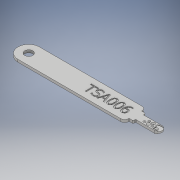
# Autodesk Inventor part: TSA006
Saved by Autodesk Inventor 2018 (Build 220112000, 112)
## iProperties
Created: 2018-08-22
Part Number: TSA006
Material: Generic
Document SubType Name: Modeling
Designer: Fatts
Density: 1 g/cm^3
Appearance: Default
Author: Fatts
Autodesk Inventor part; units mm, degrees
ref_plane "YZ Plane" through (0, 0, 0) normal (1, 0, 0) x (0, 1, 0)
ref_plane "XZ Plane" through (0, 0, 0) normal (0, 1, 0) x (-1, 0, 0)
ref_plane "XY Plane" through (0, 0, 0) normal (0, 0, 1) x (1, 0, 0)
sketch "Sketch1" plane through (0, 0, 0) normal (0, 1, 0) x (-1, 0, 0)
  line L0 (3.048, 7.366) -> (3.048, -7.366)
  line L1 (-3.048, 7.366) -> (-3.048, -7.366)
  line L2 (3.048, 0) -> (-3.048, 0) construction
  line L3 (3.048, -7.366) -> (-3.048, -7.366) construction
  arc A0 (-3.048, -7.366) -> (3.048, -7.366) centre (0, -6.7917) ccw
  line L4 (4.9022, 8.636) -> (4.9022, 10.6426)
  line L5 (-4.9022, 10.6426) -> (-4.9022, 8.636)
  line L6 (4.9022, 9.6393) -> (-4.9022, 9.6393) construction
  line L7 (0, 0) -> (0, 9.6393) construction
  line L8 (-4.0132, 7.747) -> (-3.429, 7.747)
  line L9 (3.429, 7.747) -> (4.0132, 7.747)
  arc A1 (4.0132, 7.747) -> (4.9022, 8.636) centre (4.0132, 8.636) ccw
  arc A2 (-4.9022, 8.636) -> (-4.0132, 7.747) centre (-4.0132, 8.636) ccw
  arc A3 (3.429, 7.747) -> (3.048, 7.366) centre (3.429, 7.366) ccw
  arc A4 (-3.048, 7.366) -> (-3.429, 7.747) centre (-3.429, 7.366) ccw
  line L10 (8.3947, 102.9462) -> (8.3947, 11.0236)
  line L11 (-8.3947, 102.9462) -> (-8.3947, 11.0236)
  line L12 (-8.3947, 56.9849) -> (8.3947, 56.9849) construction
  line L13 (0, 9.6393) -> (0, 56.9849) construction
  line L14 (5.2832, 11.0236) -> (8.3947, 11.0236)
  line L15 (-8.3947, 11.0236) -> (-5.2832, 11.0236)
  arc A5 (-4.9022, 10.6426) -> (-5.2832, 11.0236) centre (-5.2832, 10.6426) ccw
  arc A6 (5.2832, 11.0236) -> (4.9022, 10.6426) centre (5.2832, 10.6426) ccw
  line L16 (8.3947, 102.9462) -> (-8.3947, 102.9462)
  point P0 (4.9022, 7.747)
  point P1 (4.9022, 11.0236)
  dimension "d1" = 6.096
  dimension "d2" = 2.5273
  dimension "d3" = 7.366
  dimension "d8" = 9.8044
  dimension "d9" = 3.2766
  dimension "d10" = 0.889
  dimension "d11" = 0.381
  dimension "d12" = 16.7894
  dimension "d13" = 0.381
  dimension "d14" = 47.3456
  constraints: 34 end point, 14 point on circle, 12 tangent, 9 midpoint, 8 horizontal, 8 vertical, 7 centre point, 4 point on line, 3 equal radius, 1 coincident, 1 collinear
  measures "d1" distance between parallel lines of L0 L1
  measures "d2" distance edge to line of A0 L3
  measures "d3" distance from line of point (0, 0) L3
  measures "d8" distance of L6.start L6.end
  measures "d9" distance of point (4.902, 7.747) point (4.902, 11.024)
  measures "d10" radius of A1
  measures "d11" radius of A3
  measures "d12" distance of L12.start L12.end
  measures "d13" radius of A5
  measures "d14" distance of L7.end L13.end
extrude "MainBody" add sketch "Sketch1" along normal blind 2.02
full round fillet "EndFillet" first side at (8.3947, 0.6733, 72.3053) centre faces at (-2.7982, 0.6733, 102.9462) second side at (-8.3947, 0.6733, 41.6645)
fillet "GripFillet" radius 3.1242 2 edges at (8.3947, 1.01, 11.0236) (-8.3947, 1.01, 11.0236)
sketch "Sketch7" plane through (0, 2.02, 0) normal (0, 1, 0) x (1, 0, 0)
  line L0 (-2.4536, 5.1435) -> (2.4536, 5.1435)
  line L1 (2.4536, 5.1435) -> (2.4536, 9.8933)
  line L2 (-2.4536, 5.1435) -> (-2.4536, 9.8933)
  line L3 (-2.4536, 9.8933) -> (2.4536, 9.8933)
  line L4 (0, 0) -> (0, 5.1435) construction
  dimension "d147" = 4.9073
  dimension "d148" = 9.8933
  dimension "d149" = 4.7498
  constraints: 10 end point, 2 perpendicular, 2 vertical, 1 horizontal, 1 midpoint
  measures "d147" distance of L0.start L0.end
  measures "d148" distance from line of L3 L4.start
  measures "d149" distance of L0.end L1.end
extrude "WardingTop" cut sketch "Sketch7" against normal blind 0.41
extrude "WardingBottom" cut sketch "Sketch7" along normal blind 0.41 from surface at -2.02
sketch "Sketch2" plane through (0, 2.02, 0) normal (0, 1, 0) x (1, 0, 0)
  arc A0 (-8.3947, -94.5515) -> (8.3947, -94.5515) centre (0, -94.5515) ccw construction
  line L0 (-8.3947, -94.5515) -> (8.3947, -94.5515) construction
  circle A1 centre (0, -94.5515) radius 3.175
  point P0 (0, 0)
  dimension "d18" = 6.35
  constraints: 2 end point, 1 centre point, 1 coincident, 1 horizontal
  measures "d18" diameter of A1
extrude "RingHole" cut sketch "Sketch2" against normal through all
sketch "Sketch3" plane through (0, 2.02, 0) normal (0, 1, 0) x (1, 0, 0)
  line L0 (0, 0) -> (0, 9.8933) construction
  arc A0 (3.048, 7.366) -> (-3.048, 7.366) centre (0, 6.7917) ccw construction
  line L1 (-2.9336, 9.8933) -> (2.9336, 9.8933) construction
  circle A1 centre (1.1151, 3.4925) radius 0.889
  line L2 (3.048, -7.366) -> (3.048, 7.366) projected
  circle A2 centre (-1.1176, 5.1435) radius 0.889
  circle A3 centre (1.1151, -2.7559) radius 0.889
  circle A4 centre (-1.1176, -1.1049) radius 0.889
  point P0 (0, 9.8933)
  dimension "d21" = 1.9329
  dimension "d22" = 6.4008
  dimension "d23" = 1.778
  dimension "d24" = 1.778
  dimension "d25" = 4.7498
  dimension "d26" = 4.1656
  dimension "d27" = 1.778
  dimension "d28" = 1.9329
  dimension "d29" = 6.2484
  dimension "d30" = 1.778
  dimension "d31" = 4.1656
  dimension "d32" = 6.2484
  constraints: 4 centre point, 4 end point, 2 point on circle, 1 horizontal, 1 midpoint, 1 vertical
  measures "d21" distance from line of L2 A1.centre
  measures "d22" distance from line of L1 A1.centre
  measures "d23" diameter of A1
  measures "d24" diameter of A2
  measures "d25" distance from line of L1 A2.centre
  measures "d26" distance from line of L2 A2.centre
  measures "d27" diameter of A3
  measures "d28" distance from line of L2 A3.centre
  measures "d29" distance of A1.centre A3.centre
  measures "d30" diameter of A4
  measures "d31" distance from line of L2 A4.centre
  measures "d32" distance of A2.centre A4.centre
extrude "SmallDimpleTop" cut sketch "Sketch3" against normal blind 0.41
sketch "Sketch4" plane through (0, 2.02, 0) normal (0, 1, 0) x (1, 0, 0)
  line L0 (0, 0) -> (0, 9.8933) construction
  arc A0 (3.048, 7.366) -> (-3.048, 7.366) centre (0, 6.7917) ccw construction
  line L1 (-3.5523, 9.8933) -> (3.5523, 9.8933) construction
  circle A1 centre (1.1151, 0.3683) radius 1.3335
  line L2 (3.048, -7.366) -> (3.048, 7.366) construction
  circle A2 centre (-1.1176, 2.0193) radius 1.3335
  circle A3 centre (1.1176, 6.6167) radius 1.3335
  point P0 (0, 9.8933)
  dimension "d38" = 2.667
  dimension "d39" = 1.9329
  dimension "d40" = 9.525
  dimension "d41" = 2.667
  dimension "d42" = 4.1656
  dimension "d43" = 7.874
  dimension "d64" = 2.667
  dimension "d65" = 1.9304
  dimension "d66" = 6.2484
  constraints: 4 end point, 3 centre point, 2 point on circle, 1 horizontal, 1 midpoint, 1 vertical
  measures "d38" diameter of A1
  measures "d39" distance from line of L2 A1.centre
  measures "d40" distance from line of L1 A1.centre
  measures "d41" diameter of A2
  measures "d42" distance from line of L2 A2.centre
  measures "d43" distance from line of L1 A2.centre
  measures "d64" diameter of A3
  measures "d65" distance from line of A3.centre L2
  measures "d66" distance of A1.centre A3.centre
extrude "LargeDimpleTop" cut sketch "Sketch4" against normal blind 1.0033
sketch "Sketch5" plane through (0, 0, 0) normal (0, -1, 0) x (1, 0, 0)
  circle A0 centre (1.1151, 1.1049) radius 0.889
  circle A1 centre (-1.1176, 2.7559) radius 0.889
  circle A2 centre (1.1151, -5.1435) radius 0.889
  circle A3 centre (-1.1176, -3.4925) radius 0.889
  line L0 (0, 0) -> (0, -9.8933) construction
  arc A4 (-3.048, -7.366) -> (3.048, -7.366) centre (0, -6.7917) ccw construction
  line L1 (2.4831, -9.8933) -> (-2.4831, -9.8933) construction
  line L2 (-3.048, -7.366) -> (-3.048, 7.366) construction
  point P0 (0, -9.8933)
  dimension "d73" = 1.778
  dimension "d74" = 1.778
  dimension "d77" = 1.778
  dimension "d79" = 6.2484
  dimension "d80" = 1.778
  dimension "d82" = 6.2484
  dimension "d83" = 6.4008
  dimension "d84" = 4.7498
  dimension "d85" = 1.9304
  dimension "d86" = 4.1631
  dimension "d87" = 4.1631
  dimension "d88" = 1.9304
  constraints: 4 centre point, 4 end point, 2 point on circle, 1 horizontal, 1 midpoint, 1 vertical
  measures "d73" diameter of A0
  measures "d74" diameter of A1
  measures "d77" diameter of A2
  measures "d79" distance of A0.centre A2.centre
  measures "d80" diameter of A3
  measures "d82" distance of A1.centre A3.centre
  measures "d83" distance from line of L1 A3.centre
  measures "d84" distance from line of L1 A2.centre
  measures "d85" distance from line of L2 A3.centre
  measures "d86" distance from line of L2 A2.centre
  measures "d87" distance from line of L2 A0.centre
  measures "d88" distance from line of L2 A1.centre
extrude "SmallDimpleBottom" cut sketch "Sketch5" against normal blind 0.41
sketch "Sketch6" plane through (0, 0, 0) normal (0, -1, 0) x (1, 0, 0)
  circle A0 centre (-1.1176, -6.6167) radius 1.3335
  circle A1 centre (-1.1176, -0.3683) radius 1.3335
  circle A2 centre (1.1176, -2.0193) radius 1.3335
  line L0 (0, 0) -> (0, -9.8933) construction
  arc A3 (-3.048, -7.366) -> (3.048, -7.366) centre (0, -6.7917) ccw construction
  line L1 (3.7489, -9.8933) -> (-3.7489, -9.8933) construction
  line L2 (-3.048, -7.366) -> (-3.048, 7.366) construction
  point P0 (0, -9.8933)
  dimension "d91" = 2.667
  dimension "d92" = 2.667
  dimension "d93" = 2.667
  dimension "d95" = 1.9304
  dimension "d96" = 1.9304
  dimension "d97" = 6.2484
  dimension "d98" = 9.525
  dimension "d99" = 4.1656
  dimension "d100" = 7.874
  constraints: 4 end point, 3 centre point, 2 point on circle, 1 horizontal, 1 midpoint, 1 vertical
  measures "d91" diameter of A0
  measures "d92" diameter of A1
  measures "d93" diameter of A2
  measures "d95" distance from line of L2 A1.centre
  measures "d96" distance from line of L2 A0.centre
  measures "d97" distance of A0.centre A1.centre
  measures "d98" distance from line of L1 A1.centre
  measures "d99" distance from line of L2 A2.centre
  measures "d100" distance from line of L1 A2.centre
extrude "LargeDimpleBottom" cut sketch "Sketch6" against normal blind 1.0033
sketch "Sketch8" plane through (0, 2.02, 0) normal (0, 1, 0) x (1, 0, 0)
  line L0 (0, 0) -> (0, -49.1363) construction
  line L1 (-3.8152, -49.1363) -> (-3.8152, -14.8463) construction
  line L2 (-3.8152, -14.8463) -> (3.8152, -14.8463) construction
  line L3 (3.8152, -14.8463) -> (3.8152, -49.1363) construction
  line L4 (3.8152, -49.1363) -> (-3.8152, -49.1363) construction
  line L5 (3.6222, -46.6965) -> (-2.8051, -46.6965)
  line L6 (-2.8051, -46.6965) -> (-2.8051, -49.1422)
  line L7 (-2.8051, -49.1422) -> (-3.6676, -49.1422)
  line L8 (-3.6676, -49.1422) -> (-3.6676, -43.282)
  line L9 (-3.6676, -43.282) -> (-2.8051, -43.282)
  line L10 (-2.8051, -43.282) -> (-2.8051, -45.7277)
  line L11 (-2.8051, -45.7277) -> (3.6222, -45.7277)
  line L12 (3.6222, -45.7277) -> (3.6222, -46.6965)
  spline S0 degree 2 poles (3.7522, -40.5114) (3.7522, -41.303) (3.4214, -42.4136) (3.1851, -42.9039) knots 0 0 0 1 2 2 2
  line L13 (3.1851, -42.9039) -> (1.9682, -42.9039)
  line L14 (1.9682, -42.9039) -> (1.9682, -42.833)
  spline S1 degree 2 poles (1.9682, -42.833) (2.4171, -42.3545) (2.9134, -41.1435) (2.9134, -40.5823) knots 0 0 0 1 2 2 2
  spline S2 degree 2 poles (2.9134, -40.5823) (2.9134, -39.7789) (2.2458, -38.9578) (1.6964, -38.9578) knots 0 0 0 1 2 2 2
  spline S3 degree 2 poles (1.6964, -38.9578) (1.2593, -38.9578) (0.7158, -39.389) (0.5799, -39.8557) knots 0 0 0 1 2 2 2
  spline S4 degree 2 poles (0.5799, -39.8557) (0.4854, -40.1924) (0.3554, -40.7536) (0.2491, -41.1731) knots 0 0 0 1 2 2 2
  spline S5 degree 2 poles (0.2491, -41.1731) (0.1487, -41.5511) (-0.1526, -42.1478) (-0.3948, -42.3782) knots 0 0 0 1 2 2 2
  spline S6 degree 2 poles (-0.3948, -42.3782) (-0.637, -42.6027) (-1.2868, -42.8508) (-1.7122, -42.8508) knots 0 0 0 1 2 2 2
  spline S7 degree 2 poles (-1.7122, -42.8508) (-2.5983, -42.8508) (-3.7975, -41.4684) (-3.7975, -40.3992) knots 0 0 0 1 2 2 2
  spline S8 degree 2 poles (-3.7975, -40.3992) (-3.7975, -39.7848) (-3.5553, -38.6978) (-3.3249, -38.2311) knots 0 0 0 1 2 2 2
  line L15 (-3.3249, -38.2311) -> (-2.1671, -38.2311)
  line L16 (-2.1671, -38.2311) -> (-2.1671, -38.302)
  spline S9 degree 2 poles (-2.1671, -38.302) (-2.4861, -38.6506) (-2.9587, -39.7375) (-2.9587, -40.3342) knots 0 0 0 1 2 2 2
  spline S10 degree 2 poles (-2.9587, -40.3342) (-2.9587, -41.0076) (-2.3266, -41.8406) (-1.8126, -41.8406) knots 0 0 0 1 2 2 2
  spline S11 degree 2 poles (-1.8126, -41.8406) (-1.3518, -41.8406) (-0.8024, -41.3503) (-0.6784, -40.8895) knots 0 0 0 1 2 2 2
  spline S12 degree 2 poles (-0.6784, -40.8895) (-0.5957, -40.5823) (-0.383, -39.6903) (-0.2944, -39.3949) knots 0 0 0 1 2 2 2
  spline S13 degree 2 poles (-0.2944, -39.3949) (-0.064, -38.6447) (0.8635, -37.9476) (1.5428, -37.9476) knots 0 0 0 1 2 2 2
  spline S14 degree 2 poles (1.5428, -37.9476) (1.9741, -37.9476) (2.8011, -38.2961) (3.0906, -38.6092) knots 0 0 0 1 2 2 2
  spline S15 degree 2 poles (3.0906, -38.6092) (3.4096, -38.9578) (3.7522, -39.8439) (3.7522, -40.5114) knots 0 0 0 1 2 2 2
  line L17 (3.6222, -37.7467) -> (-3.6676, -35.2892)
  line L18 (-3.6676, -35.2892) -> (-3.6676, -34.0959)
  line L19 (-3.6676, -34.0959) -> (3.6222, -31.6384)
  line L20 (3.6222, -31.6384) -> (3.6222, -32.6604)
  line L21 (3.6222, -32.6604) -> (1.5842, -33.322)
  line L22 (1.5842, -33.322) -> (1.5842, -36.1045)
  line L23 (1.5842, -36.1045) -> (3.6222, -36.7661)
  line L24 (3.6222, -36.7661) -> (3.6222, -37.7467)
  line L25 (0.7571, -33.5879) -> (-2.6751, -34.7162)
  line L26 (-2.6751, -34.7162) -> (0.7571, -35.8386)
  line L27 (0.7571, -35.8386) -> (0.7571, -33.5879)
  spline S16 degree 2 poles (-0.0227, -26.6171) (1.9386, -26.6171) (3.7758, -27.7572) (3.7758, -28.9446) knots 0 0 0 1 2 2 2
  spline S17 degree 2 poles (3.7758, -28.9446) (3.7758, -30.1497) (1.9032, -31.2781) (-0.0167, -31.2781) knots 0 0 0 1 2 2 2
  spline S18 degree 2 poles (-0.0167, -31.2781) (-1.9898, -31.2781) (-3.8152, -30.1379) (-3.8152, -28.9446) knots 0 0 0 1 2 2 2
  spline S19 degree 2 poles (-3.8152, -28.9446) (-3.8152, -27.7454) (-1.9249, -26.6171) (-0.0227, -26.6171) knots 0 0 0 1 2 2 2
  spline S20 degree 2 poles (2.1986, -27.8695) (1.8382, -27.7277) (0.7276, -27.6095) (-0.0227, -27.6095) knots 0 0 0 1 2 2 2
  spline S21 degree 2 poles (-0.0227, -27.6095) (-0.7729, -27.6095) (-1.8776, -27.7277) (-2.2498, -27.8754) knots 0 0 0 1 2 2 2
  spline S22 degree 2 poles (-2.2498, -27.8754) (-2.6219, -28.0231) (-3.0059, -28.537) (-3.0059, -28.9446) knots 0 0 0 1 2 2 2
  spline S23 degree 2 poles (-3.0059, -28.9446) (-3.0059, -29.3522) (-2.6219, -29.878) (-2.2379, -30.0316) knots 0 0 0 1 2 2 2
  spline S24 degree 2 poles (-2.2379, -30.0316) (-1.8658, -30.1793) (-0.7315, -30.2856) (-0.0167, -30.2856) knots 0 0 0 1 2 2 2
  spline S25 degree 2 poles (-0.0167, -30.2856) (0.7512, -30.2856) (1.7791, -30.1911) (2.1808, -30.0375) knots 0 0 0 1 2 2 2
  spline S26 degree 2 poles (2.1808, -30.0375) (2.5589, -29.8957) (2.9665, -29.37) (2.9665, -28.9446) knots 0 0 0 1 2 2 2
  spline S27 degree 2 poles (2.9665, -28.9446) (2.9665, -28.5429) (2.5825, -28.0171) (2.1986, -27.8695) knots 0 0 0 1 2 2 2
  spline S28 degree 2 poles (-0.0227, -21.1468) (1.9386, -21.1468) (3.7758, -22.2869) (3.7758, -23.4743) knots 0 0 0 1 2 2 2
  spline S29 degree 2 poles (3.7758, -23.4743) (3.7758, -24.6794) (1.9032, -25.8078) (-0.0167, -25.8078) knots 0 0 0 1 2 2 2
  spline S30 degree 2 poles (-0.0167, -25.8078) (-1.9898, -25.8078) (-3.8152, -24.6676) (-3.8152, -23.4743) knots 0 0 0 1 2 2 2
  spline S31 degree 2 poles (-3.8152, -23.4743) (-3.8152, -22.2751) (-1.9249, -21.1468) (-0.0227, -21.1468) knots 0 0 0 1 2 2 2
  spline S32 degree 2 poles (2.1986, -22.3992) (1.8382, -22.2574) (0.7276, -22.1392) (-0.0227, -22.1392) knots 0 0 0 1 2 2 2
  spline S33 degree 2 poles (-0.0227, -22.1392) (-0.7729, -22.1392) (-1.8776, -22.2574) (-2.2498, -22.4051) knots 0 0 0 1 2 2 2
  spline S34 degree 2 poles (-2.2498, -22.4051) (-2.6219, -22.5528) (-3.0059, -23.0667) (-3.0059, -23.4743) knots 0 0 0 1 2 2 2
  spline S35 degree 2 poles (-3.0059, -23.4743) (-3.0059, -23.8819) (-2.6219, -24.4077) (-2.2379, -24.5613) knots 0 0 0 1 2 2 2
  spline S36 degree 2 poles (-2.2379, -24.5613) (-1.8658, -24.709) (-0.7315, -24.8153) (-0.0167, -24.8153) knots 0 0 0 1 2 2 2
  spline S37 degree 2 poles (-0.0167, -24.8153) (0.7512, -24.8153) (1.7791, -24.7208) (2.1808, -24.5672) knots 0 0 0 1 2 2 2
  spline S38 degree 2 poles (2.1808, -24.5672) (2.5589, -24.4254) (2.9665, -23.8997) (2.9665, -23.4743) knots 0 0 0 1 2 2 2
  spline S39 degree 2 poles (2.9665, -23.4743) (2.9665, -23.0726) (2.5825, -22.5468) (2.1986, -22.3992) knots 0 0 0 1 2 2 2
  spline S40 degree 2 poles (1.2593, -15.6056) (1.8205, -15.6056) (2.7716, -15.9778) (3.0906, -16.2908) knots 0 0 0 1 2 2 2
  spline S41 degree 2 poles (3.0906, -16.2908) (3.4273, -16.6158) (3.7758, -17.431) (3.7758, -17.9213) knots 0 0 0 1 2 2 2
  spline S42 degree 2 poles (3.7758, -17.9213) (3.7758, -18.4116) (3.445, -19.2209) (3.1142, -19.5281) knots 0 0 0 1 2 2 2
  spline S43 degree 2 poles (3.1142, -19.5281) (2.7184, -19.9062) (1.3892, -20.3315) (0.4204, -20.3315) knots 0 0 0 1 2 2 2
  spline S44 degree 2 poles (0.4204, -20.3315) (-0.5307, -20.3315) (-2.0607, -19.9417) (-2.6278, -19.534) knots 0 0 0 1 2 2 2
  spline S45 degree 2 poles (-2.6278, -19.534) (-3.1831, -19.1382) (-3.8034, -17.8859) (-3.8034, -17.0647) knots 0 0 0 1 2 2 2
  spline S46 degree 2 poles (-3.8034, -17.0647) (-3.8034, -16.8225) (-3.7562, -16.3972) (-3.703, -16.2377) knots 0 0 0 1 2 2 2
  line L28 (-3.703, -16.2377) -> (-2.7637, -16.2377)
  line L29 (-2.7637, -16.2377) -> (-2.7637, -16.279)
  spline S47 degree 2 poles (-2.7637, -16.279) (-2.8346, -16.4149) (-2.9587, -16.9111) (-2.9587, -17.1947) knots 0 0 0 1 2 2 2
  spline S48 degree 2 poles (-2.9587, -17.1947) (-2.9587, -18.1044) (-1.7299, -19.2209) (-0.5248, -19.3273) knots 0 0 0 1 2 2 2
  spline S49 degree 2 poles (-0.5248, -19.3273) (-0.767, -18.9787) (-1.0328, -18.2462) (-1.0328, -17.8091) knots 0 0 0 1 2 2 2
  spline S50 degree 2 poles (-1.0328, -17.8091) (-1.0328, -17.3837) (-0.8615, -16.7457) (-0.6016, -16.3972) knots 0 0 0 1 2 2 2
  spline S51 degree 2 poles (-0.6016, -16.3972) (-0.3003, -15.9955) (0.6331, -15.6056) (1.2593, -15.6056) knots 0 0 0 1 2 2 2
  spline S52 degree 2 poles (1.3006, -16.598) (0.8517, -16.598) (0.2432, -16.8343) (0.0305, -17.0943) knots 0 0 0 1 2 2 2
  spline S53 degree 2 poles (0.0305, -17.0943) (-0.1231, -17.2892) (-0.2235, -17.7736) (-0.2235, -18.0276) knots 0 0 0 1 2 2 2
  spline S54 degree 2 poles (-0.2235, -18.0276) (-0.2235, -18.3703) (-0.0167, -19.0142) (0.1782, -19.3273) knots 0 0 0 1 2 2 2
  spline S55 degree 2 poles (0.1782, -19.3273) (0.2845, -19.3332) (0.4854, -19.345) (0.639, -19.345) knots 0 0 0 1 2 2 2
  spline S56 degree 2 poles (0.639, -19.345) (1.3951, -19.345) (2.3226, -19.0496) (2.5648, -18.8251) knots 0 0 0 1 2 2 2
  spline S57 degree 2 poles (2.5648, -18.8251) (2.7952, -18.6184) (2.9783, -18.1694) (2.9783, -17.9154) knots 0 0 0 1 2 2 2
  spline S58 degree 2 poles (2.9783, -17.9154) (2.9783, -17.3247) (2.1395, -16.598) (1.3006, -16.598) knots 0 0 0 1 2 2 2
  dimension "d144" = 34.29
  dimension "d145" = 7.6305
  dimension "d146" = 49.1363
  constraints: 2 end point, 2 vertical, 1 midpoint, 2 other
  measures "d144" distance of L1.start L1.end
  measures "d145" distance of L3.end L1.start
  measures "d146" distance from line of L0.start L4
extrude "LogoTop" cut sketch "Sketch8" against normal blind 0.508
sketch "Sketch9" plane through (0, 0, 0) normal (0, -1, 0) x (1, 0, 0)
  line L0 (4.0729, 49.1363) -> (4.0729, 14.8463) construction
  line L1 (4.0729, 14.8463) -> (-4.0729, 14.8463) construction
  line L2 (-4.0729, 14.8463) -> (-4.0729, 49.1363) construction
  line L3 (-4.0729, 49.1363) -> (4.0729, 49.1363) construction
  line L4 (0, 0) -> (0, 49.1363) construction
  line L5 (-3.3646, 46.6965) -> (3.0627, 46.6965)
  line L6 (3.0627, 46.6965) -> (3.0627, 49.1422)
  line L7 (3.0627, 49.1422) -> (3.9252, 49.1422)
  line L8 (3.9252, 49.1422) -> (3.9252, 43.282)
  line L9 (3.9252, 43.282) -> (3.0627, 43.282)
  line L10 (3.0627, 43.282) -> (3.0627, 45.7277)
  line L11 (3.0627, 45.7277) -> (-3.3646, 45.7277)
  line L12 (-3.3646, 45.7277) -> (-3.3646, 46.6965)
  spline S0 degree 2 poles (-3.4946, 40.5114) (-3.4946, 41.303) (-3.1638, 42.4136) (-2.9275, 42.9039) knots 0 0 0 1 2 2 2
  line L13 (-2.9275, 42.9039) -> (-1.7105, 42.9039)
  line L14 (-1.7105, 42.9039) -> (-1.7105, 42.833)
  spline S1 degree 2 poles (-1.7105, 42.833) (-2.1595, 42.3545) (-2.6557, 41.1435) (-2.6557, 40.5823) knots 0 0 0 1 2 2 2
  spline S2 degree 2 poles (-2.6557, 40.5823) (-2.6557, 39.7789) (-1.9882, 38.9578) (-1.4388, 38.9578) knots 0 0 0 1 2 2 2
  spline S3 degree 2 poles (-1.4388, 38.9578) (-1.0016, 38.9578) (-0.4582, 39.389) (-0.3223, 39.8557) knots 0 0 0 1 2 2 2
  spline S4 degree 2 poles (-0.3223, 39.8557) (-0.2278, 40.1924) (-0.0978, 40.7536) (0.0085, 41.1731) knots 0 0 0 1 2 2 2
  spline S5 degree 2 poles (0.0085, 41.1731) (0.109, 41.5511) (0.4102, 42.1478) (0.6524, 42.3782) knots 0 0 0 1 2 2 2
  spline S6 degree 2 poles (0.6524, 42.3782) (0.8947, 42.6027) (1.5445, 42.8508) (1.9698, 42.8508) knots 0 0 0 1 2 2 2
  spline S7 degree 2 poles (1.9698, 42.8508) (2.8559, 42.8508) (4.0551, 41.4684) (4.0551, 40.3992) knots 0 0 0 1 2 2 2
  spline S8 degree 2 poles (4.0551, 40.3992) (4.0551, 39.7848) (3.8129, 38.6978) (3.5825, 38.2311) knots 0 0 0 1 2 2 2
  line L15 (3.5825, 38.2311) -> (2.4247, 38.2311)
  line L16 (2.4247, 38.2311) -> (2.4247, 38.302)
  spline S9 degree 2 poles (2.4247, 38.302) (2.7437, 38.6506) (3.2163, 39.7375) (3.2163, 40.3342) knots 0 0 0 1 2 2 2
  spline S10 degree 2 poles (3.2163, 40.3342) (3.2163, 41.0076) (2.5842, 41.8406) (2.0702, 41.8406) knots 0 0 0 1 2 2 2
  spline S11 degree 2 poles (2.0702, 41.8406) (1.6095, 41.8406) (1.0601, 41.3503) (0.936, 40.8895) knots 0 0 0 1 2 2 2
  spline S12 degree 2 poles (0.936, 40.8895) (0.8533, 40.5823) (0.6406, 39.6903) (0.552, 39.3949) knots 0 0 0 1 2 2 2
  spline S13 degree 2 poles (0.552, 39.3949) (0.3216, 38.6447) (-0.6058, 37.9476) (-1.2852, 37.9476) knots 0 0 0 1 2 2 2
  spline S14 degree 2 poles (-1.2852, 37.9476) (-1.7164, 37.9476) (-2.5435, 38.2961) (-2.8329, 38.6092) knots 0 0 0 1 2 2 2
  spline S15 degree 2 poles (-2.8329, 38.6092) (-3.152, 38.9578) (-3.4946, 39.8439) (-3.4946, 40.5114) knots 0 0 0 1 2 2 2
  line L17 (-3.3646, 37.7467) -> (3.9252, 35.2892)
  line L18 (3.9252, 35.2892) -> (3.9252, 34.0959)
  line L19 (3.9252, 34.0959) -> (-3.3646, 31.6384)
  line L20 (-3.3646, 31.6384) -> (-3.3646, 32.6604)
  line L21 (-3.3646, 32.6604) -> (-1.3265, 33.322)
  line L22 (-1.3265, 33.322) -> (-1.3265, 36.1045)
  line L23 (-1.3265, 36.1045) -> (-3.3646, 36.7661)
  line L24 (-3.3646, 36.7661) -> (-3.3646, 37.7467)
  line L25 (-0.4995, 33.5879) -> (2.9327, 34.7162)
  line L26 (2.9327, 34.7162) -> (-0.4995, 35.8386)
  line L27 (-0.4995, 35.8386) -> (-0.4995, 33.5879)
  spline S16 degree 2 poles (0.2803, 26.6171) (-1.681, 26.6171) (-3.5182, 27.7572) (-3.5182, 28.9446) knots 0 0 0 1 2 2 2
  spline S17 degree 2 poles (-3.5182, 28.9446) (-3.5182, 30.1497) (-1.6456, 31.2781) (0.2744, 31.2781) knots 0 0 0 1 2 2 2
  spline S18 degree 2 poles (0.2744, 31.2781) (2.2475, 31.2781) (4.0729, 30.1379) (4.0729, 28.9446) knots 0 0 0 1 2 2 2
  spline S19 degree 2 poles (4.0729, 28.9446) (4.0729, 27.7454) (2.1825, 26.6171) (0.2803, 26.6171) knots 0 0 0 1 2 2 2
  spline S20 degree 2 poles (-1.9409, 27.8695) (-1.5806, 27.7277) (-0.47, 27.6095) (0.2803, 27.6095) knots 0 0 0 1 2 2 2
  spline S21 degree 2 poles (0.2803, 27.6095) (1.0305, 27.6095) (2.1352, 27.7277) (2.5074, 27.8754) knots 0 0 0 1 2 2 2
  spline S22 degree 2 poles (2.5074, 27.8754) (2.8796, 28.0231) (3.2635, 28.537) (3.2635, 28.9446) knots 0 0 0 1 2 2 2
  spline S23 degree 2 poles (3.2635, 28.9446) (3.2635, 29.3522) (2.8796, 29.878) (2.4956, 30.0316) knots 0 0 0 1 2 2 2
  spline S24 degree 2 poles (2.4956, 30.0316) (2.1234, 30.1793) (0.9892, 30.2856) (0.2744, 30.2856) knots 0 0 0 1 2 2 2
  spline S25 degree 2 poles (0.2744, 30.2856) (-0.4936, 30.2856) (-1.5215, 30.1911) (-1.9232, 30.0375) knots 0 0 0 1 2 2 2
  spline S26 degree 2 poles (-1.9232, 30.0375) (-2.3013, 29.8957) (-2.7089, 29.37) (-2.7089, 28.9446) knots 0 0 0 1 2 2 2
  spline S27 degree 2 poles (-2.7089, 28.9446) (-2.7089, 28.5429) (-2.3249, 28.0171) (-1.9409, 27.8695) knots 0 0 0 1 2 2 2
  spline S28 degree 2 poles (0.2803, 21.1468) (-1.681, 21.1468) (-3.5182, 22.2869) (-3.5182, 23.4743) knots 0 0 0 1 2 2 2
  spline S29 degree 2 poles (-3.5182, 23.4743) (-3.5182, 24.6794) (-1.6456, 25.8078) (0.2744, 25.8078) knots 0 0 0 1 2 2 2
  spline S30 degree 2 poles (0.2744, 25.8078) (2.2475, 25.8078) (4.0729, 24.6676) (4.0729, 23.4743) knots 0 0 0 1 2 2 2
  spline S31 degree 2 poles (4.0729, 23.4743) (4.0729, 22.2751) (2.1825, 21.1468) (0.2803, 21.1468) knots 0 0 0 1 2 2 2
  spline S32 degree 2 poles (-1.9409, 22.3992) (-1.5806, 22.2574) (-0.47, 22.1392) (0.2803, 22.1392) knots 0 0 0 1 2 2 2
  spline S33 degree 2 poles (0.2803, 22.1392) (1.0305, 22.1392) (2.1352, 22.2574) (2.5074, 22.4051) knots 0 0 0 1 2 2 2
  spline S34 degree 2 poles (2.5074, 22.4051) (2.8796, 22.5528) (3.2635, 23.0667) (3.2635, 23.4743) knots 0 0 0 1 2 2 2
  spline S35 degree 2 poles (3.2635, 23.4743) (3.2635, 23.8819) (2.8796, 24.4077) (2.4956, 24.5613) knots 0 0 0 1 2 2 2
  spline S36 degree 2 poles (2.4956, 24.5613) (2.1234, 24.709) (0.9892, 24.8153) (0.2744, 24.8153) knots 0 0 0 1 2 2 2
  spline S37 degree 2 poles (0.2744, 24.8153) (-0.4936, 24.8153) (-1.5215, 24.7208) (-1.9232, 24.5672) knots 0 0 0 1 2 2 2
  spline S38 degree 2 poles (-1.9232, 24.5672) (-2.3013, 24.4254) (-2.7089, 23.8997) (-2.7089, 23.4743) knots 0 0 0 1 2 2 2
  spline S39 degree 2 poles (-2.7089, 23.4743) (-2.7089, 23.0726) (-2.3249, 22.5468) (-1.9409, 22.3992) knots 0 0 0 1 2 2 2
  spline S40 degree 2 poles (-1.0016, 15.6056) (-1.5628, 15.6056) (-2.5139, 15.9778) (-2.8329, 16.2908) knots 0 0 0 1 2 2 2
  spline S41 degree 2 poles (-2.8329, 16.2908) (-3.1697, 16.6158) (-3.5182, 17.431) (-3.5182, 17.9213) knots 0 0 0 1 2 2 2
  spline S42 degree 2 poles (-3.5182, 17.9213) (-3.5182, 18.4116) (-3.1874, 19.2209) (-2.8566, 19.5281) knots 0 0 0 1 2 2 2
  spline S43 degree 2 poles (-2.8566, 19.5281) (-2.4608, 19.9062) (-1.1316, 20.3315) (-0.1628, 20.3315) knots 0 0 0 1 2 2 2
  spline S44 degree 2 poles (-0.1628, 20.3315) (0.7883, 20.3315) (2.3184, 19.9417) (2.8855, 19.534) knots 0 0 0 1 2 2 2
  spline S45 degree 2 poles (2.8855, 19.534) (3.4408, 19.1382) (4.0611, 17.8859) (4.0611, 17.0647) knots 0 0 0 1 2 2 2
  spline S46 degree 2 poles (4.0611, 17.0647) (4.0611, 16.8225) (4.0138, 16.3972) (3.9606, 16.2377) knots 0 0 0 1 2 2 2
  line L28 (3.9606, 16.2377) -> (3.0213, 16.2377)
  line L29 (3.0213, 16.2377) -> (3.0213, 16.279)
  spline S47 degree 2 poles (3.0213, 16.279) (3.0922, 16.4149) (3.2163, 16.9111) (3.2163, 17.1947) knots 0 0 0 1 2 2 2
  spline S48 degree 2 poles (3.2163, 17.1947) (3.2163, 18.1044) (1.9875, 19.2209) (0.7824, 19.3273) knots 0 0 0 1 2 2 2
  spline S49 degree 2 poles (0.7824, 19.3273) (1.0246, 18.9787) (1.2905, 18.2462) (1.2905, 17.8091) knots 0 0 0 1 2 2 2
  spline S50 degree 2 poles (1.2905, 17.8091) (1.2905, 17.3837) (1.1191, 16.7457) (0.8592, 16.3972) knots 0 0 0 1 2 2 2
  spline S51 degree 2 poles (0.8592, 16.3972) (0.5579, 15.9955) (-0.3754, 15.6056) (-1.0016, 15.6056) knots 0 0 0 1 2 2 2
  spline S52 degree 2 poles (-1.043, 16.598) (-0.594, 16.598) (0.0144, 16.8343) (0.2271, 17.0943) knots 0 0 0 1 2 2 2
  spline S53 degree 2 poles (0.2271, 17.0943) (0.3807, 17.2892) (0.4811, 17.7736) (0.4811, 18.0276) knots 0 0 0 1 2 2 2
  spline S54 degree 2 poles (0.4811, 18.0276) (0.4811, 18.3703) (0.2744, 19.0142) (0.0794, 19.3273) knots 0 0 0 1 2 2 2
  spline S55 degree 2 poles (0.0794, 19.3273) (-0.0269, 19.3332) (-0.2278, 19.345) (-0.3814, 19.345) knots 0 0 0 1 2 2 2
  spline S56 degree 2 poles (-0.3814, 19.345) (-1.1375, 19.345) (-2.065, 19.0496) (-2.3072, 18.8251) knots 0 0 0 1 2 2 2
  spline S57 degree 2 poles (-2.3072, 18.8251) (-2.5376, 18.6184) (-2.7207, 18.1694) (-2.7207, 17.9154) knots 0 0 0 1 2 2 2
  spline S58 degree 2 poles (-2.7207, 17.9154) (-2.7207, 17.3247) (-1.8818, 16.598) (-1.043, 16.598) knots 0 0 0 1 2 2 2
  dimension "d141" = 49.1363
  dimension "d142" = 8.1457
  dimension "d143" = 34.29
  constraints: 2 end point, 2 vertical, 1 midpoint, 2 other
  measures "d141" distance of L4.start L4.end
  measures "d142" distance of L2.end L0.start
  measures "d143" distance of L1.end L2.end
extrude "LogoBottom" cut sketch "Sketch9" against normal blind 0.508
chamfer "SmallDimpleChamfer" distance 0.41 angle 45 8 edges at (1.1151, 0.41, -4.2545) (-2.0066, 0.41, -3.4925) (0.2261, 0.41, 1.1049) (-2.0066, 0.41, 2.7559) (-1.1176, 1.61, -4.2545) (0.2261, 1.61, -3.4925) (-2.0066, 1.61, 1.1049) (0.2261, 1.61, 2.7559)
chamfer "LargeDimpleChamfer" distance 1.0033 angle 45 4 edges at (-2.4511, 1.0167, -2.0193) (-0.2184, 1.0167, -0.3683) (-2.4511, 1.0033, -0.3683) (-0.2159, 1.0033, -2.0193)
chamfer "LargeWardingDimpleChamfer" distance 0.5933 angle 45 2 edges at (-2.4511, 1.0033, -6.6167) (-0.2159, 1.0167, -6.6167)
body "Solid1"
